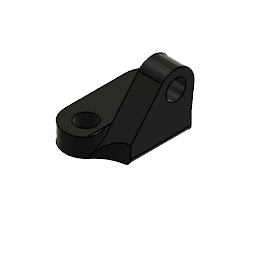
Dribbler attachment (Autodesk Fusion 360 design; units mm, degrees)
part number: 2026-05-02-21-13-35-798
Autodesk Fusion 360 part; units mm, degrees
sketch "Sketch1" plane through (0, 0, 0) normal (0, 1, 0) x (1, 0, 0)
  circle A0 centre (0, 0) radius 1.65
  circle A1 centre (0, 0) radius 3.5
  line L0 (0, 0) -> (0, -10)
  circle A2 centre (0, -10) radius 1.65
  circle A3 centre (0, -10) radius 3.5
  line L1 (0, 0) -> (-3.5, 0) construction
  line L2 (-3.5, 0) -> (-3.5, -10)
  line L3 (3.5, 0) -> (3.5, -10)
  dimension "d1" = 3.3
  dimension "d2" = 7
  dimension "d3" = 10
  dimension "d4" = 3.3
  dimension "d5" = 7
  constraint coincident A0.centre A1.centre
  constraint vertical L0
  constraint coincident L0.end A2.centre
  constraint concentric A2 A3
  constraint coincident A1 L1.end
  constraint perpendicular L0 L1
  constraint coincident A3 L2.end
  constraint tangent A3 L2
  constraint coincident A1 L3.start
  constraint coincident A3 L3.end
  constraint tangent A3 L3
  constraint parallel L2 L3
  measures "d1" diameter of A0
  measures "d2" diameter of A1
  measures "d3" distance of A0.centre L0.end
  measures "d4" diameter of A2
  measures "d5" diameter of A3
extrude "Extrude1" add sketch "Sketch1" along normal blind 3
sketch "Sketch2" plane through (3.5, 0, 0) normal (1, 0, 0) x (0, 0, -1)
  line L0 (-10, 0) -> (0, 0)
  line L1 (0, 0) -> (0, 3)
  line L2 (0, 3) -> (-10, 3)
  line L3 (-10, 3) -> (-10, 0)
  line L4 (-5, 3) -> (-2.5, 7.3301)
  line L5 (-5, 3) -> (0, 3) construction
  circle A0 centre (-2.5, 7.3301) radius 1.65
  circle A1 centre (-2.5, 7.3301) radius 3
  line L6 (-10, 3) -> (-4.8071, 9.2477)
  line L7 (0, 3) -> (0.4785, 6.9713)
  dimension "d8" = 60
  dimension "d9" = 5
  dimension "d10" = 3.3
  dimension "d11" = 6
  constraint horizontal L5
  constraint midpoint L2 L4.start
  constraint coincident L4.end A0.centre
  constraint coincident L2.end L3.start
  constraint coincident A1 L6.end
  constraint tangent A1 L6
  constraint coincident L1.end L2.start
  constraint coincident A1 L7.end
  constraint tangent A1 L7
  measures "d8" angle of L4 L5
  measures "d9" distance of L4.start L4.end
  measures "d10" diameter of A0
  measures "d11" diameter of A1
extrude "Extrude2" add sketch "Sketch2" along normal blind 3.9
fillet "Fillet1" radius 1 1 edges at (3.5, 3, 5)
fillet "Fillet2" radius 1 1 edges at (7.4, 0, 5)
fillet "Fillet3" radius 6 1 edges at (3.5, 1.5, 10)
fillet "Fillet4" radius 20 1 edges at (3.5, 1.5, 0)
equation "d12 = 3.00 mm + 0.9 mm"
